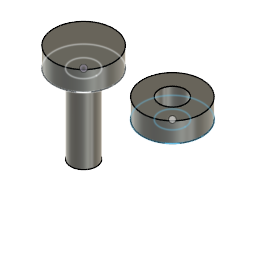
joystick mount (Autodesk Fusion 360 design; units mm, degrees)
part number: 2026-07-03-13-31-37-306
Autodesk Fusion 360 part; units mm, degrees
sketch "Sketch1" plane through (0, 0, 0) normal (0, 0, 1) x (1, 0, 0)
  circle A0 centre (0, 0) radius 1.3
  circle A1 centre (0, 0) radius 3
  circle A2 centre (9, 0) radius 1.3
  circle A3 centre (9, 0) radius 3
  dimension "d1" = 2.6
  dimension "d2" = 6
  dimension "d7" = 2.6
  dimension "d8" = 6
  constraint coincident A0.centre A1.centre
  constraint concentric A0 A1
  constraint concentric A2 A3
  measures "d1" diameter of A0
  measures "d2" diameter of A1
  measures "d7" diameter of A2
  measures "d8" diameter of A3
extrude "Extrude1" add sketch "Sketch1" along normal blind 2 contours A0 | A1 makes body 1
extrude "Extrude2" add sketch "Sketch1" against normal blind 8 separate body contours A0 makes body 2
extrude "Extrude3" add sketch "Sketch1" along normal blind 2 separate body contours A3 makes body 3
